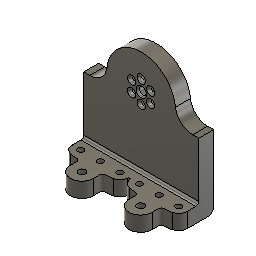
Holder2 v12 (Autodesk Fusion 360 archive; units mm, degrees)
design "HolderBase"
Autodesk Fusion 360 part; units mm, degrees
sketch "Sketch1" plane through (0, 20, -46.4489) normal (0, 0, 1) x (-1, 0, 0)
  circle A0 centre (0.9947, -83.8573) radius 3
  circle A1 centre (0.9947, -83.8573) radius 6
  circle A2 centre (0.9947, -83.8573) radius 6
  circle A3 centre (0.9947, -83.8573) radius 3.05
  circle A4 centre (0.9947, -83.8573) radius 30
  line L0 (50.9947, -10.8573) -> (-49.0053, -10.8573)
  line L1 (-49.0053, -10.8573) -> (-49.0053, -83.8573)
  line L2 (-49.0053, -83.8573) -> (50.9947, -83.8573)
  line L3 (50.9947, -83.8573) -> (50.9947, -10.8573)
  line L4 (50.9947, -10.8573) -> (-49.0053, -83.8573) construction
  line L5 (-49.0053, -10.8573) -> (50.9947, -83.8573) construction
  line L6 (-49.0053, -23.8573) -> (50.9947, -23.8573)
  line L7 (-49.0053, -73.8573) -> (50.9947, -73.8573)
  point P0 (0.9947, -47.3573)
  dimension "d70" = 60
  dimension "d111" = 12
  dimension "d208" = 50
  dimension "d209" = 100
  dimension "d210" = 13
  dimension "d6" = 6.1
  dimension "d18" = 60
  dimension "d19" = 10
  constraint concentric A0 A2
  constraint concentric A2 A3
  constraint concentric A2 A4
  constraint horizontal L0
  constraint perpendicular L0 L1
  constraint parallel L0 L2
  constraint parallel L1 L3
  constraint coincident L4 P0
  constraint coincident L5 P0
  constraint coincident A0.centre L2
  constraint coincident L1 L6.start
  constraint coincident L3 L6.end
  constraint perpendicular L3 L6
  constraint coincident L1 L7.start
  constraint coincident L3 L7.end
  constraint perpendicular L3 L7
  measures "d70" diameter of A4
  measures "d111" diameter of A2
  measures "d208" distance of A0.centre L1
  measures "d209" distance of L0.start L0.end
  measures "d210" distance of L0 L6
  measures "d6" diameter of A3
  measures "d18" distance of L2 L6
  measures "d19" distance of L2 L7
extrude "Extrude1" add sketch "Sketch1" along normal blind 13 contours A1 A2 A3 L2 | A1 A2 A3 L2 | A1 A2 A4 L2 | A1 A2 A4 L2 L7 | A4 L7 | A4 L1 L3 L6 L7
extrude "Extrude6" add sketch "Sketch1" along normal blind 53 contours L0 L1 L3 L6
sketch "Sketch2" plane through (0, 43.8573, 0) normal (0, 1, 0) x (-1, 0, 0)
  line L0 (-49.0053, -33.4489) -> (50.9947, -33.4489)
  line L1 (50.9947, -33.4489) -> (50.9947, 6.5511)
  line L2 (50.9947, 6.5511) -> (-49.0053, 6.5511)
  line L3 (-49.0053, 6.5511) -> (-49.0053, -33.4489)
  line L4 (0.9947, -100) -> (0.9947, 25)
  circle A0 centre (43.4947, -23.4489) radius 2.55
  circle A1 centre (43.4947, -23.4489) radius 7.5
  line L5 (50.9947, -33.4489) -> (-49.0053, -33.4489)
  line L6 (-49.0053, -33.4489) -> (-49.0053, 6.5511)
  line L7 (-49.0053, 6.5511) -> (50.9947, 6.5511)
  line L8 (50.9947, 6.5511) -> (50.9947, -33.4489)
  circle A2 centre (26.4947, -23.4489) radius 7.5
  circle A3 centre (26.4947, -23.4489) radius 2.55
  circle A4 centre (9.4947, -23.4489) radius 7.5
  circle A5 centre (9.4947, -23.4489) radius 2.55
  line L9 (50.9947, -23.4489) -> (0.9947, -23.4489)
  circle A6 centre (-41.5053, -23.4489) radius 7.5
  circle A7 centre (-41.5053, -23.4489) radius 2.55
  line L10 (-49.0053, -23.4489) -> (0.9947, -23.4489)
  circle A8 centre (-24.5053, -23.4489) radius 7.5
  circle A9 centre (-24.5053, -23.4489) radius 2.55
  circle A10 centre (-7.5053, -23.4489) radius 7.5
  circle A11 centre (-7.5053, -23.4489) radius 2.55
  circle A12 centre (26.4947, -7.4489) radius 3.05
  circle A13 centre (26.4947, -7.4489) radius 10
  line L11 (50.9947, -7.4489) -> (0.9947, -7.4489)
  spline S0 degree 5 poles (36.4947, -7.4489) (36.5142, -7.782) (36.5365, -8.4586) (36.5197, -9.5049) (36.4281, -10.9328) (36.3682, -12.6126) (36.5621, -14.004) (37.1816, -14.9597) (38.3015, -15.4385) (39.8392, -15.5688) (41.6323, -15.5639) (43.1209, -15.6414) (44.1969, -15.8336) (44.8868, -16.0334) (45.2248, -16.1512) knots 0 0 0 0 0 0 0.1 0.2 0.3 0.4 0.5 0.6 0.7 0.8 0.9 1 1 1 1 1 1
  line L12 (26.4947, -23.4489) -> (26.4947, -7.4489) construction
  spline S1 degree 5 poles (16.4947, -7.4489) (16.4752, -7.782) (16.453, -8.4586) (16.4698, -9.5049) (16.5613, -10.9328) (16.6213, -12.6126) (16.4274, -14.004) (15.8079, -14.9597) (14.688, -15.4385) (13.1502, -15.5688) (11.3571, -15.5639) (9.8686, -15.6414) (8.7925, -15.8336) (8.1027, -16.0334) (7.7647, -16.1512) knots 0 0 0 0 0 0 0.1 0.2 0.3 0.4 0.5 0.6 0.7 0.8 0.9 1 1 1 1 1 1
  line L13 (36.3896, -5.6527) -> (36.5999, -9.2451)
  line L14 (43.5142, -15.5551) -> (46.9353, -16.7473)
  line L15 (16.5999, -5.6527) -> (16.3896, -9.2451)
  line L16 (9.4753, -15.5551) -> (6.0541, -16.7473)
  circle A14 centre (-24.5053, -7.4489) radius 10
  circle A15 centre (-24.5053, -7.4489) radius 3.05
  line L17 (-49.0053, -7.4489) -> (0.9947, -7.4489)
  spline S2 degree 5 poles (-14.5053, -7.4489) (-14.4858, -7.782) (-14.4635, -8.4586) (-14.4803, -9.5049) (-14.5719, -10.9328) (-14.6318, -12.6126) (-14.4379, -14.004) (-13.8184, -14.9597) (-12.6985, -15.4385) (-11.1608, -15.5688) (-9.3677, -15.5639) (-7.8791, -15.6414) (-6.8031, -15.8336) (-6.1132, -16.0334) (-5.7752, -16.1512) knots 0 0 0 0 0 0 0.1 0.2 0.3 0.4 0.5 0.6 0.7 0.8 0.9 1 1 1 1 1 1
  line L18 (-14.6104, -5.6527) -> (-14.4001, -9.2451)
  line L19 (-7.4858, -15.5551) -> (-4.0647, -16.7473)
  spline S3 degree 5 poles (-34.5053, -7.4489) (-34.5248, -7.782) (-34.547, -8.4586) (-34.5302, -9.5049) (-34.4387, -10.9328) (-34.3787, -12.6126) (-34.5726, -14.004) (-35.1921, -14.9597) (-36.312, -15.4385) (-37.8498, -15.5688) (-39.6429, -15.5639) (-41.1314, -15.6414) (-42.2075, -15.8336) (-42.8973, -16.0334) (-43.2353, -16.1512) knots 0 0 0 0 0 0 0.1 0.2 0.3 0.4 0.5 0.6 0.7 0.8 0.9 1 1 1 1 1 1
  line L20 (-34.4001, -5.6527) -> (-34.6104, -9.2451)
  line L21 (-41.5247, -15.5551) -> (-44.9459, -16.7473)
  line L22 (45.2248, -16.1512) -> (36.4947, -7.4489) construction
  line L23 (40.8598, -11.8001) -> (26.4947, -23.4489) construction
  point P0 (0.9947, -46.4489)
  point P1 (37.2113, -14.7587)
  point P2 (15.7782, -14.7587)
  point P3 (-13.7887, -14.7587)
  point P4 (-35.2218, -14.7587)
  dimension "d232" = 5.1
  dimension "d233" = 15
  dimension "d234" = 10
  dimension "d237" = -34
  dimension "d238" = 0
  dimension "d239" = 6.1
  dimension "d240" = 20
  dimension "d241" = 16
  constraint perpendicular L2 L4
  constraint coincident L4 P0
  constraint concentric A0 A1
  constraint horizontal L5
  constraint vertical L6
  constraint horizontal L7
  constraint vertical L8
  constraint coincident L2.end L3.start
  constraint coincident L0.end L1.start
  constraint tangent A1 L8
  constraint coincident L8 L9.start
  constraint coincident A1 L9.start
  constraint coincident L4 L9.end
  constraint perpendicular L4 L9
  constraint symmetric L4 A0 A7
  constraint symmetric L4 A1 A6
  constraint symmetric L4 A2 A8
  constraint symmetric L4 A3 A9
  constraint symmetric L4 A4 A10
  constraint symmetric L4 A5 A11
  constraint symmetric L4 L9.start L10.start
  constraint symmetric L4 L9.end L10.end
  constraint concentric A12 A13
  constraint coincident L8 L11.start
  constraint coincident L4 L11.end
  constraint perpendicular L4 L11
  constraint coincident A13 S0.start
  constraint coincident L11 S0.start
  constraint coincident A1 S0.end
  constraint coincident A2.centre A3.centre
  constraint coincident A12.centre A13.centre
  constraint perpendicular L11 L12
  constraint midpoint S0.start L13
  constraint midpoint S0.end L14
  constraint symmetric S0.start L12 S1.start
  constraint symmetric P1 L12 P2
  constraint symmetric S0.end L12 S1.end
  constraint symmetric L12 L13.start L15.start
  constraint symmetric L12 L13.end L15.end
  constraint symmetric L12 L14.start L16.start
  constraint symmetric L12 L14.end L16.end
  constraint symmetric L4 A12 A15
  constraint symmetric L4 A13 A14
  constraint symmetric L4 L11.start L17.start
  constraint symmetric L4 L11.end L17.end
  constraint symmetric L4 S0.start S3.start
  constraint symmetric L4 P1 P4
  constraint symmetric L4 S0.end S3.end
  constraint symmetric L4 S1.start S2.start
  constraint symmetric L4 P2 P3
  constraint symmetric L4 S1.end S2.end
  constraint symmetric L4 L13.start L20.start
  constraint symmetric L4 L13.end L20.end
  constraint symmetric L4 L14.start L21.start
  constraint symmetric L4 L14.end L21.end
  constraint symmetric L4 L15.start L18.start
  constraint symmetric L4 L15.end L18.end
  constraint symmetric L4 L16.start L19.start
  constraint symmetric L4 L16.end L19.end
  constraint coincident A12.centre L11
  constraint midpoint L22 L23.start
  constraint coincident P1 L23
  measures "d232" diameter of A0
  measures "d233" diameter of A1
  measures "d234" distance of A0.centre L5
  measures "d239" diameter of A12
  measures "d240" diameter of A13
  measures "d241" distance of L9 L11
extrude "Extrude9" cut sketch "Sketch2" against normal up to surface (13 mm away) contours L3 L6 A6 L17 S3 | L4 L10 A10 L17 S2 | L4 A4 L9 L11 S1 | L2 L3 L4 L6 L7 A14 L17 | A7 L10 | A7 L10 | L1 A1 L8 L11 S0 | L1 L2 L4 L7 L8 A13 L11 | A0 L9 | A0 L9 | A5 L9 | A5 L9 | L10 A11 | L10 A11 | A15 L17 | A15 L17 | L10 A9 | L10 A9 | A12 L11 | A12 L11 | A3 L9 | A3 L9
fillet "Fillet3" radius 1 2 edges at (-1.9947, 37.3573, -23.4489) (0.0053, 37.3573, -23.4489)
fillet "Fillet4" radius 3 6 edges at (43.8827, 30.8573, -24.371) (26.8827, 30.8573, -24.371) (9.8827, 30.8573, -24.371) (-7.1173, 30.8573, -24.371) (-24.1173, 30.8573, -24.371) (-41.1173, 30.8573, -24.371)
fillet "Fillet5" radius 3.5 2 edges at (27.3489, 30.8573, -8.5519) (-23.6511, 30.8573, -8.5519)
sketch "Sketch3" plane through (0, 0, -46.4489) normal (0, 0, -1) x (-1, 0, 0)
  line L0 (-49.0053, 93.8573) -> (-49.0053, 30.8573)
  line L1 (-49.0053, 30.8573) -> (50.9947, 30.8573)
  line L2 (50.9947, 30.8573) -> (50.9947, 93.8573)
  line L3 (50.9947, 93.8573) -> (29.279, 93.8573)
  arc A0 (29.279, 93.8573) -> (-27.2895, 93.8573) centre (0.9947, 103.8573) ccw
  line L4 (-27.2895, 93.8573) -> (-49.0053, 93.8573)
  circle A1 centre (0.9947, 103.8573) radius 9.525 construction
  line L5 (0.9947, 117.0724) -> (0.9947, 116)
  line L6 (0.9947, 116) -> (0.9947, 91) construction
  circle A2 centre (0.9947, 113.3823) radius 1.55
  circle A3 centre (-7.2542, 108.6198) radius 1.55
  circle A4 centre (-7.2542, 99.0948) radius 1.55
  circle A5 centre (0.9947, 94.3323) radius 1.55
  circle A6 centre (9.2436, 99.0948) radius 1.55
  circle A7 centre (9.2436, 108.6198) radius 1.55
  circle A8 centre (0.9947, 103.8573) radius 3.05
  dimension "d8" = 19.05
  dimension "d9" = 3.1
  dimension "d11" = 360
  constraint concentric A1 A8
  constraint vertical L5
  constraint parallel L5 L6
  constraint coincident A0.centre L6
  constraint coincident L6 A2.centre
  constraint coincident A1 A2.centre
  measures "d8" diameter of A1
  measures "d9" diameter of A2
extrude "Extrude10" cut sketch "Sketch3" against normal blind 15 contours A2 | A3 | A4 | A5 | A6 | A7
fillet "Fillet6" radius 2.1 6 edges at (8.6993, 98.5343, -33.4489) (0.4504, 93.7718, -33.4489) (-7.7985, 98.5343, -33.4489) (-7.7985, 108.0593, -33.4489) (0.4504, 112.8218, -33.4489) (8.6993, 108.0593, -33.4489)
fillet "Fillet6" radius 1.5 1 edges at (1.8489, 102.7544, -33.4489)
fillet "Fillet7" radius 15 2 edges at (27.2895, 93.8573, -39.9489) (-29.279, 93.8573, -39.9489)
fillet "Fillet8" radius 2.5 1 edges at (-0.9947, 43.8573, -33.4489)
fillet "Fillet9" radius 5 1 edges at (-0.9947, 30.8573, -46.4489)
equation "d209 = d208 * 2"
equation "d18 = 1 cm + 4 cm + 1 cm"
